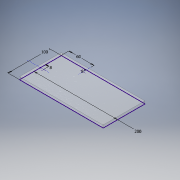
# Autodesk Inventor part: BT004_trajan20_21
Saved by Autodesk Inventor 2022.2 (Build 262287000, 287)
## iProperties
Company: HTBLA Kaindorf
RuleStatus: InUse
Created: 2022-08-07
Part Number: BT004_trajan20_21
Project: Zeichenmaschine_v2
Material: Acryl
Description: Hauptplatte unten
Document SubType Name: Modeling
Designer: trajan20
Density: 1.188 g/cm^3
Appearance: Transparent - farblos
Mass: 142.536 g
Surface Area: 435.725 cm^2
Volume: 119.979 cm^3
AfterDocNew0: iProperties-Editor_aufrufen
Author: jan
Keywords: 2021
Autodesk Inventor part; units mm, degrees
ref_plane "YZ Plane" through (0, 0, 0) normal (1, 0, 0) x (0, 1, 0)
ref_plane "XZ Plane" through (0, 0, 0) normal (0, 1, 0) x (-1, 0, 0)
ref_plane "XY Plane" through (0, 0, 0) normal (0, 0, 1) x (1, 0, 0)
sketch "Skizze4" plane through (0, 0, 0) normal (0, 0, 1) x (1, 0, 0)
  line L0 (0, 0) -> (-100, 0)
  line L1 (-100, 0) -> (-100, 200)
  line L2 (-100, 200) -> (0, 200)
  line L3 (0, 200) -> (0, 0)
  line L4 (-50, 22.6255) -> (-50, -31.1035) construction
  line L5 (-111.0989, 60) -> (-81.531, 60) construction
  point P0 (-50, 8)
  point P1 (-92, 60)
  point P2 (-50, 0)
  dimension "d6" = 100
  dimension "d7" = 200
  dimension "d20" = 8
  dimension "d21" = 8
  dimension "d31" = 60
  constraints: 12 end point, 3 perpendicular, 3 point on line, 2 horizontal, 2 parallel, 1 midpoint, 1 vertical
  measures "d6" distance between parallel lines of L1 L3
  measures "d7" distance between parallel lines of L2 L0
  measures "d20" distance from line of point (-92, 60) L1
  measures "d21" distance from line of L0 point (-50, 8)
  measures "d31" distance between parallel lines of L0 L5
extrude "Extrusion3" add sketch "Skizze4" along normal blind 6
ref_plane "Arbeitsebene1" through (0, 100, 0) normal (0, -1, 0) x (1, 0, 0)
ref_plane "Arbeitsebene2" through (-50, 200, 0) normal (-1, 0, 0) x (0, -1, 0)
fillet "Rundung2" radius 2 4 edges at (0, 0, 3) (-100, 0, 3) (-100, 200, 3) (0, 200, 3)
